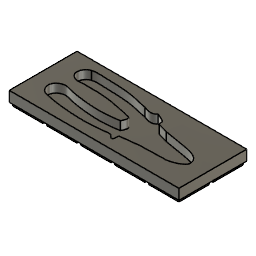
wire strippers gridfinity module (Autodesk Fusion 360 design; units mm, degrees)
Autodesk Fusion 360 part; units mm, degrees
sketch "Sketch1" plane through (0, 0, 0) normal (0, 0, 1) x (1, 0, 0)
  line L0 (20.75, -20.75) -> (-20.75, -20.75)
  line L1 (-20.75, -20.75) -> (-20.75, 20.75)
  line L2 (-20.75, 20.75) -> (20.75, 20.75)
  line L3 (20.75, 20.75) -> (20.75, -20.75)
  line L4 (20.75, -20.75) -> (-20.75, 20.75) construction
  line L5 (-20.75, -20.75) -> (20.75, 20.75) construction
  dimension "d1" = 41.5
  dimension "d2" = 41.5
  constraint horizontal L0
  constraint perpendicular L0 L1
  constraint parallel L0 L2
  constraint parallel L1 L3
  constraint coincident L4 origin
  constraint coincident L5 origin
  measures "d1" distance of L1.end L2.end
  measures "d2" distance of L0.end L1.end
extrude "Extrude1" add sketch "Sketch1" along normal blind 7 makes body 1
sketch "Sketch2" plane through (0, -20.75, 0) normal (0, -1, 0) x (1, 0, 0)
  line L0 (-20.75, 0) -> (20.75, 0)
  line L1 (20.75, 0) -> (20.75, 7)
  line L2 (20.75, 7) -> (-20.75, 7)
  line L3 (-20.75, 7) -> (-20.75, 0)
  line L4 (-20.75, 0) -> (-17.8, 0) construction
  line L5 (-17.8, 0) -> (-18.6, 0) construction
  line L6 (17.8, 0) -> (18.6, 0.8)
  line L7 (18.6, 0.8) -> (18.6, 2.6)
  line L8 (18.6, 2.6) -> (20.75, 4.75)
  line L9 (-17.8, 0) -> (-18.6, 0.8)
  line L10 (-17.8, 0) -> (-9.0611, 0) construction
  line L11 (-18.6, 0.8) -> (-18.6, 2.6)
  line L12 (-18.6, 2.6) -> (-20.75, 4.75)
  constraint coincident L0.start L3.end
  constraint perpendicular L3 L4
  constraint parallel L0 L5
  constraint coincident L1 L8.end
  constraint horizontal L10
  constraint perpendicular L5 L11
  constraint coincident L3 L12.end
sketch "Sketch3" plane through (20.75, 0, 0) normal (1, 0, 0) x (0, 1, 0)
  line L0 (-20.75, 0) -> (20.75, 0)
  line L1 (20.75, 0) -> (20.75, 7)
  line L2 (20.75, 7) -> (-20.75, 7)
  line L3 (-20.75, 7) -> (-20.75, 0)
  line L4 (-17.8, 0) -> (-18.6, 0.8)
  line L5 (-18.6, 0.8) -> (-18.6, 2.6)
  line L6 (-18.6, 2.6) -> (-20.75, 4.75)
  line L7 (20.75, 0) -> (17.8, 0) construction
  line L8 (17.8, 0) -> (18.6, 0) construction
  line L9 (17.8, 0) -> (18.6, 0.8)
  line L10 (18.6, 0.8) -> (18.6, 2.6)
  line L11 (18.6, 2.6) -> (20.75, 4.75)
  constraint coincident L3 L6.end
  constraint coincident L0.end L1.start
  constraint perpendicular L1 L7
  constraint perpendicular L1 L8
  constraint perpendicular L7 L10
  constraint coincident L1 L11.end
extrude "Extrude2" cut sketch "Sketch2" along normal mid plane 50 contours L0 L3 L9 L11 L12 | L0 L1 L6 L7 L8 bodies 1
extrude "Extrude3" cut 2 faces at (20.0333, 4.25, 2.45) (-20.0333, 4.25, 2.45) along direction (0, -1, 0) mid plane 100 on bodies 1 bodies 1
extrude "Extrude4" cut sketch "Sketch3" along normal mid plane 100 contours L0 L3 L4 L5 L6 | L0 L1 L9 L10 L11 bodies 1
copy_body "CopyPasteBodies1" bodies 1 makes body 2
move_body "Move1" bodies 2 to x (1, 0, 0) y (0, 1, 0) z (0, 0, 1) at (41.5, 0, 0)
copy_body "CopyPasteBodies2" bodies 2 makes body 3
move_body "Move2" bodies 3 to x (1, 0, 0) y (0, 1, 0) z (0, 0, 1) at (41.5, 0, 0)
move_body "Move3" bodies 1 to x (1, 0, 0) y (0, 1, 0) z (0, 0, 1) at (-80, 0, 0)
move_body "Move4" bodies 2 to x (1, 0, 0) y (0, 1, 0) z (0, 0, 1) at (-80, 0, 0)
move_body "Move5" bodies 3 to x (1, 0, 0) y (0, 1, 0) z (0, 0, 1) at (-80, 0, 0)
copy_body "CopyPasteBodies3" bodies 3 makes body 4
move_body "Move6" bodies 4 to x (1, 0, 0) y (0, 1, 0) z (0, 0, 1) at (41.5, 0, 0)
copy_body "CopyPasteBodies4" bodies 4 makes body 5
move_body "Move7" bodies 5 to x (1, 0, 0) y (0, 1, 0) z (0, 0, 1) at (41.5, 0, 0)
combine "Combine1" operation add target body 1 tool bodies 3 4 5 2
move_body "Move8" bodies 1 to x (1, 0, 0) y (0, 1, 0) z (0, 0, 1) at (-5, 0, 0)
move_body "Move9" bodies 1 to x (1, 0, 0) y (0, 1, 0) z (0, 0, 1) at (0, -10, 0)
copy_body "CopyPasteBodies5" bodies 1 makes body 6
move_body "Move10" bodies 6 to x (1, 0, 0) y (0, 1, 0) z (0, 0, 1) at (0, -41.5, 0)
combine "Combine2" operation add target body 1 tool bodies 6
move_body "Move11" bodies 1 to x (1, 0, 0) y (0, 1, 0) z (0, 0, 1) at (0, 5, 0)
sketch "Sketch4" plane through (0, 0, 0) normal (0, 0, 1) x (1, 0, 0)
  spline S0 degree 5 poles (-76.3948, 4.03) (-76.5195, 4.0227) (-76.7711, 3.9962) (-77.1553, 3.9216) (-77.6811, 3.7522) (-78.3589, 3.425) (-79.052, 2.9877) (-79.7492, 2.4523) (-80.4319, 1.8391) (-81.0786, 1.1716) (-81.6692, 0.4719) (-82.1887, -0.2442) (-82.6328, -0.9728) (-83.0082, -1.7234) (-83.326, -2.5116) (-83.5957, -3.3531) (-83.819, -4.2578) (-83.9835, -5.2226) (-84.0655, -6.2335) (-84.0371, -7.2695) (-83.8718, -8.3059) (-83.5504, -9.3181) (-83.0676, -10.2855) (-82.4328, -11.1923) (-81.6638, -12.0264) (-80.7842, -12.7791) (-79.8191, -13.4446) (-78.7909, -14.019) (-77.716, -14.5001) (-76.6052, -14.8869) (-75.4652, -15.1793) (-74.5325, -15.3379) (-73.8219, -15.4147) (-73.3433, -15.4472) (-73.1027, -15.4588) knots 0 0 0 0 0 0 0.033333 0.066667 0.1 0.133333 0.166667 0.2 0.233333 0.266667 0.3 0.333333 0.366667 0.4 0.433333 0.466667 0.5 0.533333 0.566667 0.6 0.633333 0.666667 0.7 0.733333 0.766667 0.8 0.833333 0.866667 0.9 0.933333 0.966667 1 1 1 1 1 1
  spline S1 degree 5 poles (-73.1027, -15.4588) (-72.9023, -15.429) (-72.5067, -15.3716) (-71.9289, -15.2918) (-71.1902, -15.1984) (-70.319, -15.1034) (-69.4962, -15.0303) (-68.7127, -14.9786) (-67.9499, -14.9464) (-67.1802, -14.9303) (-66.3725, -14.9266) (-65.4964, -14.9311) (-64.5275, -14.9404) (-63.4523, -14.9521) (-62.2646, -14.9647) (-60.9634, -14.9771) (-59.8329, -14.9866) (-58.9355, -14.9934) (-58.3155, -14.9978) (-58, -15) knots 0 0 0 0 0 0 0.066667 0.133333 0.2 0.266667 0.333333 0.4 0.466667 0.533333 0.6 0.666667 0.733333 0.8 0.866667 0.933333 1 1 1 1 1 1
  line L0 (-58, -15) -> (-52.4288, -15)
  spline S2 degree 5 poles (-52.4288, -15) (-52.3214, -14.9925) (-52.0973, -14.9792) (-51.7335, -14.9648) (-51.1926, -14.9567) (-50.4237, -14.965) (-49.5643, -14.9916) (-48.6213, -15.0359) (-47.608, -15.0963) (-46.5426, -15.1707) (-45.445, -15.2566) (-44.3352, -15.3513) (-43.231, -15.4525) (-42.1451, -15.5578) (-41.0845, -15.6655) (-40.0522, -15.7744) (-39.0479, -15.8834) (-38.0699, -15.9918) (-37.1156, -16.0991) (-36.1832, -16.2049) (-35.2712, -16.3092) (-34.5574, -16.3912) (-34.0306, -16.452) (-33.6833, -16.4922) (-33.5105, -16.5122) knots 0 0 0 0 0 0 0.05 0.1 0.15 0.2 0.25 0.3 0.35 0.4 0.45 0.5 0.55 0.6 0.65 0.7 0.75 0.8 0.85 0.9 0.95 1 1 1 1 1 1
  spline S3 degree 5 poles (-33.5105, -16.5122) (-33.3513, -16.518) (-33.0353, -16.5333) (-32.569, -16.5683) (-31.9624, -16.6386) (-31.2271, -16.7652) (-30.5075, -16.9271) (-29.7889, -17.1172) (-29.0463, -17.3239) (-28.2513, -17.533) (-27.3811, -17.7319) (-26.4253, -17.9122) (-25.3963, -18.0737) (-24.3285, -18.2245) (-23.2655, -18.3763) (-22.2499, -18.5404) (-21.3124, -18.7248) (-20.4608, -18.929) (-19.6712, -19.1419) (-18.9021, -19.3479) (-18.1077, -19.533) (-17.2499, -19.6902) (-16.3136, -19.8272) (-15.3064, -19.9637) (-14.2488, -20.123) (-13.1683, -20.3256) (-12.0914, -20.5827) (-11.0362, -20.8874) (-10.0082, -21.2132) (-9.007, -21.5261) (-8.0308, -21.7942) (-7.0819, -21.998) (-6.1712, -22.1407) (-5.324, -22.2593) (-4.5753, -22.4142) (-3.9631, -22.6759) (-3.5238, -23.113) (-3.2846, -23.7784) (-3.2641, -24.7082) (-3.4741, -25.9258) (-3.9211, -27.4443) (-4.4703, -28.9046) (-4.9903, -30.1384) (-5.3848, -31.0226) (-5.5941, -31.48) knots 0 0 0 0 0 0 0.025 0.05 0.075 0.1 0.125 0.15 0.175 0.2 0.225 0.25 0.275 0.3 0.325 0.35 0.375 0.4 0.425 0.45 0.475 0.5 0.525 0.55 0.575 0.6 0.625 0.65 0.675 0.7 0.725 0.75 0.775 0.8 0.825 0.85 0.875 0.9 0.925 0.95 0.975 1 1 1 1 1 1
  spline S4 degree 5 poles (-5.5941, -31.48) (-5.8708, -31.5202) (-6.4336, -31.6014) (-7.3058, -31.7261) (-8.5251, -31.8981) (-10.1436, -32.122) (-11.8586, -32.3531) (-13.674, -32.5878) (-15.5963, -32.8203) (-17.6342, -33.0426) (-19.7972, -33.2455) (-22.0955, -33.4193) (-24.5382, -33.5542) (-27.1333, -33.6413) (-29.8862, -33.6731) (-32.7979, -33.6434) (-35.8637, -33.5478) (-39.0712, -33.3838) (-42.399, -33.1509) (-45.8144, -32.8507) (-49.2725, -32.4875) (-52.7134, -32.068) (-56.0638, -31.6019) (-59.2466, -31.1007) (-62.1897, -30.578) (-64.835, -30.0486) (-67.1469, -29.5285) (-69.1214, -29.0339) (-70.7944, -28.5815) (-72.2531, -28.1874) (-73.6126, -27.8701) (-74.9853, -27.6547) (-76.4548, -27.5754) (-78.0441, -27.6809) (-79.7251, -28.023) (-81.435, -28.6438) (-83.0897, -29.5641) (-84.5991, -30.7678) (-85.8785, -32.2032) (-86.8561, -33.7995) (-87.4827, -35.48) (-87.7391, -37.175) (-87.6468, -38.8376) (-87.2581, -40.4391) (-86.6398, -41.9582) (-85.8599, -43.3742) (-84.9717, -44.6552) (-84.0075, -45.7615) (-82.9805, -46.6635) (-81.8862, -47.3535) (-80.7014, -47.8643) (-79.3927, -48.2582) (-77.9276, -48.6039) (-76.2858, -48.9569) (-74.4691, -49.3406) (-72.4942, -49.7555) (-70.3884, -50.187) (-68.1827, -50.6138) (-65.9073, -51.0155) (-63.5847, -51.3814) (-61.2303, -51.7092) (-58.8528, -52.002) (-56.4552, -52.2668) (-54.0349, -52.5113) (-51.5845, -52.7428) (-49.0925, -52.9643) (-46.5445, -53.1756) (-43.9254, -53.3734) (-41.2214, -53.5521) (-38.422, -53.7048) (-35.522, -53.8238) (-32.5232, -53.9012) (-29.4373, -53.9298) (-26.2847, -53.904) (-23.0937, -53.8197) (-19.8992, -53.6758) (-16.7415, -53.4743) (-13.6649, -53.2214) (-10.717, -52.9276) (-7.9469, -52.6088) (-5.4051, -52.2871) (-3.1374, -51.9909) (-1.1783, -51.7549) (0.4568, -51.6215) (1.7778, -51.6391) (2.8293, -51.8664) (3.6904, -52.3604) (4.4508, -53.1263) (5.1857, -54.0537) (5.9438, -54.9244) (6.7557, -55.5072) (7.4604, -55.6222) (8.0222, -55.4915) (8.4115, -55.3076) (8.6099, -55.1914) knots 0 0 0 0 0 0 0.01111111 0.02222222 0.03333333 0.04444444 0.05555556 0.06666667 0.07777778 0.08888889 0.1 0.11111111 0.12222222 0.13333333 0.14444444 0.15555556 0.16666667 0.17777778 0.18888889 0.2 0.21111111 0.22222222 0.23333333 0.24444444 0.25555556 0.26666667 0.27777778 0.28888889 0.3 0.31111111 0.32222222 0.33333333 0.34444444 0.35555556 0.36666667 0.37777778 0.38888889 0.4 0.41111111 0.42222222 0.43333333 0.44444444 0.45555556 0.46666667 0.47777778 0.48888889 0.5 0.51111111 0.52222222 0.53333333 0.54444444 0.55555556 0.56666667 0.57777778 0.58888889 0.6 0.61111111 0.62222222 0.63333333 0.64444444 0.65555556 0.66666667 0.67777778 0.68888889 0.7 0.71111111 0.72222222 0.73333333 0.74444444 0.75555556 0.76666667 0.77777778 0.78888889 0.8 0.81111111 0.82222222 0.83333333 0.84444444 0.85555556 0.86666667 0.87777778 0.88888889 0.9 0.91111111 0.92222222 0.93333333 0.94444444 0.95555556 0.96666667 0.97777778 0.98888889 1 1 1 1 1 1
  spline S5 degree 5 poles (8.6099, -55.1914) (8.666, -55.1856) (8.7729, -55.1679) (8.9182, -55.1229) (9.0813, -55.0258) (9.2345, -54.8429) (9.3386, -54.6002) (9.3979, -54.3027) (9.421, -53.96) (9.4188, -53.5844) (9.4031, -53.1896) (9.3848, -52.7881) (9.3725, -52.3899) (9.3704, -52.0003) (9.3789, -51.6201) (9.3958, -51.2474) (9.4174, -50.8786) (9.4396, -50.5095) (9.4591, -50.1367) (9.4738, -49.758) (9.4826, -49.3724) (9.4844, -49.0579) (9.4829, -48.8186) (9.4805, -48.6575) (9.479, -48.5766) knots 0 0 0 0 0 0 0.05 0.1 0.15 0.2 0.25 0.3 0.35 0.4 0.45 0.5 0.55 0.6 0.65 0.7 0.75 0.8 0.85 0.9 0.95 1 1 1 1 1 1
  line L1 (9.479, -48.5766) -> (32.4471, -45.8617)
  line L2 (32.4471, -45.8617) -> (61, -45)
  spline S6 degree 5 poles (61, -45) (61.1296, -45.0372) (61.403, -45.1004) (61.8554, -45.1618) (62.5437, -45.1768) (63.5413, -45.0871) (64.6635, -44.8976) (65.8826, -44.6274) (67.1595, -44.3025) (68.4525, -43.9491) (69.7242, -43.5862) (70.9494, -43.2199) (72.124, -42.8356) (73.2583, -42.4059) (74.3686, -41.9029) (75.4696, -41.3069) (76.5654, -40.6198) (77.6443, -39.8691) (78.6827, -39.0919) (79.6483, -38.3208) (80.5031, -37.5713) (81.2059, -36.8231) (81.7196, -36.029) (82.0246, -35.1474) (82.1281, -34.1653) (82.079, -33.131) (81.9443, -32.1225) (81.7806, -31.2113) (81.6058, -30.4224) (81.3778, -29.7079) (81.0309, -28.9925) (80.5046, -28.2119) (79.7751, -27.3523) (78.8437, -26.4344) (77.7279, -25.4985) (76.452, -24.5905) (75.0363, -23.7453) (73.4922, -22.9796) (71.8252, -22.2977) (70.0356, -21.6934) (68.1206, -21.1534) (66.0752, -20.6609) (63.8936, -20.1978) (61.5714, -19.7488) (59.1052, -19.3015) (56.4925, -18.8462) (53.7318, -18.3752) (50.8222, -17.883) (47.7633, -17.3656) (44.555, -16.8205) (41.1977, -16.2462) (38.3928, -15.7628) (36.2224, -15.3867) (34.7457, -15.1299) (34, -15) knots 0 0 0 0 0 0 0.02 0.04 0.06 0.08 0.1 0.12 0.14 0.16 0.18 0.2 0.22 0.24 0.26 0.28 0.3 0.32 0.34 0.36 0.38 0.4 0.42 0.44 0.46 0.48 0.5 0.52 0.54 0.56 0.58 0.6 0.62 0.64 0.66 0.68 0.7 0.72 0.74 0.76 0.78 0.8 0.82 0.84 0.86 0.88 0.9 0.92 0.94 0.96 0.98 1 1 1 1 1 1
  spline S7 degree 5 poles (34, -15) (33.5238, -14.8653) (32.5713, -14.596) (31.1426, -14.1919) (29.2377, -13.6532) (26.8565, -12.9798) (24.9516, -12.4411) (23.5229, -12.0371) (22.5705, -11.7677) (22.0942, -11.6331) knots 0 0 0 0 0 0 0.2 0.4 0.6 0.8 1 1 1 1 1 1
  spline S8 degree 5 poles (22.0942, -11.6331) (22.061, -11.6017) (21.9956, -11.5333) (21.9008, -11.4133) (21.7808, -11.2183) (21.6423, -10.9123) (21.516, -10.5402) (21.4024, -10.0992) (21.3012, -9.5917) (21.2111, -9.0235) (21.1312, -8.4008) (21.0745, -7.8632) (21.0358, -7.4395) (21.0117, -7.148) (21, -7) knots 0 0 0 0 0 0 0.1 0.2 0.3 0.4 0.5 0.6 0.7 0.8 0.9 1 1 1 1 1 1
  spline S9 degree 5 poles (21, -7) (20.9845, -6.9361) (20.9335, -6.8032) (20.7974, -6.5889) (20.4944, -6.2725) (19.9036, -5.8235) (19.092, -5.3187) (18.0649, -4.7596) (16.8418, -4.1511) (15.4455, -3.4989) (13.8977, -2.8085) (12.5516, -2.2289) (11.4858, -1.78) (10.7507, -1.4746) (10.377, -1.3203) knots 0 0 0 0 0 0 0.1 0.2 0.3 0.4 0.5 0.6 0.7 0.8 0.9 1 1 1 1 1 1
  spline S10 degree 5 poles (10.377, -1.3203) (10.208, -1.5522) (9.8569, -1.9955) (9.2917, -2.5996) (8.4595, -3.2813) (7.2803, -3.9143) (5.9526, -4.3132) (4.4691, -4.4667) (2.8338, -4.3809) (1.0592, -4.0754) (-0.841, -3.572) (-2.452, -3.0262) (-3.7078, -2.5418) (-4.5658, -2.1861) (-5, -2) knots 0 0 0 0 0 0 0.1 0.2 0.3 0.4 0.5 0.6 0.7 0.8 0.9 1 1 1 1 1 1
  spline S11 degree 5 poles (-5, -2) (-5.1724, -1.986) (-5.5337, -1.9515) (-6.1253, -1.8806) (-7.0138, -1.7476) (-8.2858, -1.5186) (-9.7044, -1.2312) (-11.2381, -0.8945) (-12.8484, -0.5206) (-14.5014, -0.1227) (-16.1779, 0.2876) (-17.8863, 0.702) (-19.6577, 1.1156) (-21.5331, 1.525) (-23.5522, 1.9273) (-25.7426, 2.3186) (-28.1074, 2.6927) (-30.6281, 3.0414) (-33.2721, 3.3567) (-35.9982, 3.6313) (-38.7632, 3.8602) (-41.5275, 4.042) (-44.2619, 4.1802) (-46.9518, 4.2841) (-49.5929, 4.366) (-52.1868, 4.4393) (-54.738, 4.5162) (-57.2489, 4.605) (-59.7169, 4.7088) (-62.1297, 4.8219) (-64.4647, 4.9304) (-66.6936, 5.0156) (-68.7865, 5.0567) (-70.7148, 5.0334) (-72.4552, 4.9291) (-73.994, 4.7337) (-75.0589, 4.5008) (-75.7634, 4.2824) (-76.1913, 4.1174) (-76.3948, 4.03) knots 0 0 0 0 0 0 0.028571 0.057143 0.085714 0.114286 0.142857 0.171429 0.2 0.228571 0.257143 0.285714 0.314286 0.342857 0.371429 0.4 0.428571 0.457143 0.485714 0.514286 0.542857 0.571429 0.6 0.628571 0.657143 0.685714 0.714286 0.742857 0.771429 0.8 0.828571 0.857143 0.885714 0.914286 0.942857 0.971429 1 1 1 1 1 1
  point P0 (-79, 3)
  point P1 (-82, 0)
  point P2 (-83.6372, -3.5636)
  point P3 (-83.725, -8.6992)
  point P4 (-79.7746, -13.4397)
  point P5 (-69, -15)
  point P6 (-65.5091, -14.9321)
  point P7 (-49.444, -15)
  point P8 (-43.65, -15.4149)
  point P9 (-38, -16)
  point P10 (-30.438, -16.9512)
  point P11 (-26.8683, -17.8244)
  point P12 (-21.4398, -18.7069)
  point P13 (-17.7966, -19.5848)
  point P14 (-12.4415, -20.5066)
  point P15 (-7, -22)
  point P16 (-3.8683, -22.8244)
  point P17 (-12.2484, -32.4018)
  point P18 (-23.9329, -33.5123)
  point P19 (-48.1711, -32.5949)
  point P20 (-69.3191, -28.9737)
  point P21 (-75.2096, -27.67)
  point P22 (-82.2107, -29.1185)
  point P23 (-87.4736, -35.8299)
  point P24 (-86.2665, -42.5895)
  point P25 (-82.6452, -46.8385)
  point P26 (-78.0101, -48.5766)
  point P27 (-67.9189, -50.6528)
  point P28 (-53.2408, -52.5842)
  point P29 (-34.6518, -53.8395)
  point P30 (-9.8825, -52.8256)
  point P31 (1.4157, -51.6668)
  point P32 (4.1196, -52.8256)
  point P33 (6.3889, -55.1914)
  point P34 (9.3342, -54.5638)
  point P35 (9.3825, -52.6807)
  point P36 (9.4307, -50.6528)
  point P37 (64, -45)
  point P38 (69.8859, -43.5343)
  point P39 (75.1827, -41.4477)
  point P40 (80, -38)
  point P41 (82, -35)
  point P42 (81.8037, -31.3757)
  point P43 (81, -29)
  point P44 (77, -25)
  point P45 (65.4719, -20.5413)
  point P46 (21.4923, -10.4292)
  point P47 (19.486, -5.5738)
  point P48 (5.4414, -4.3299)
  point P49 (-8.4427, -1.4808)
  point P50 (-15, 0)
  point P51 (-24, 2)
  point P52 (-41, 4)
  point P53 (-58.4815, 4.6586)
  point P54 (-71, 5)
  constraint horizontal L0
sketch "Sketch5" plane through (0, 0, 7) normal (0, 0, 1) x (-1, 0, 0)
  line L0 (-101.75, -15.75) -> (105.75, -15.75)
  line L1 (105.75, -15.75) -> (105.75, 67.25)
  line L2 (105.75, 67.25) -> (-101.75, 67.25)
  line L3 (-101.75, 67.25) -> (-101.75, -15.75)
  line L4 (105.75, -15.75) -> (-101.75, -15.75)
  line L5 (-101.75, -15.75) -> (-101.75, 67.25)
  line L6 (-101.75, 67.25) -> (105.75, 67.25)
  line L7 (105.75, 67.25) -> (105.75, -15.75)
  constraint horizontal L4
  constraint vertical L5
  constraint horizontal L6
  constraint vertical L7
  constraint coincident L2.end L3.start
  constraint coincident L0.end L1.start
extrude "Extrude5" add sketch "Sketch5" along normal blind 10.5 bodies 1
move_body "Move12" bodies 1 to x (1, 0, 0) y (0, 1, 0) z (0, 0, 1) at (0, 0, -7)
extrude "Extrude6" cut sketch "Sketch4" along normal blind 10.5 bodies 1
